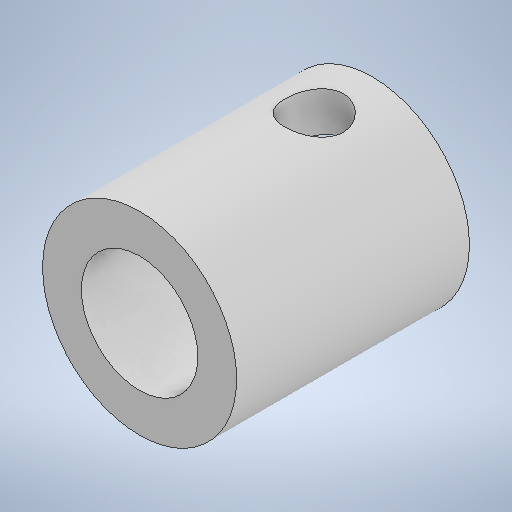
# Autodesk Inventor part: entretoise moteur cremaillere
Saved by Autodesk Inventor 2025.2 (Build 292293000, 293)
## iProperties
Created: 2025-03-30
Part Number: entretoise moteur cremaillere
Material: Générique
Document SubType Name: Modeling
Designer: enezl
Density: 1 g/cm^3
Appearance: Par défaut
Author: enezl
Autodesk Inventor part; units mm, degrees
ref_plane "YZ Plane" through (0, 0, 0) normal (1, 0, 0) x (0, 1, 0)
ref_plane "XY Plane" through (0, 0, 0) normal (0, 0, 1) x (1, 0, 0)
sketch "Esquisse1" plane through (0, 0, 0) normal (1, 0, 0) x (0, 1, 0)
  line L0 (5, 6) -> (3, 6)
  line L1 (3, 6) -> (3, -6)
  line L2 (3, -6) -> (5, -6)
  line L3 (5, -6) -> (5, 6)
  line L4 (5, 6) -> (3, -6) construction
  line L5 (3, 6) -> (5, -6) construction
  line L6 (0, 12.4388) -> (0, -12.4388)
  line L7 (0, 0) -> (14.0159, 0) construction
  point P0 (4, 0)
  dimension "d0" = 6
  dimension "d1" = 10
  dimension "d2" = 12
  constraints: 16 end point, 3 midpoint, 2 horizontal, 2 parallel, 1 coincident, 1 perpendicular, 1 point on line, 1 vertical
  measures "d0" diameter of L1 L6
  measures "d1" diameter of L3 L6
  measures "d2" distance of L2.end L0.start
revolve "Révolution1" add sketch "Esquisse1" angle 360 about axis through (0, 0, 12.4388) along (0, 0, -1)
ref_plane "Plan de construction1" through (0, 5, 0) normal (0, 1, 0) x (-1, 0, 0)
sketch "Esquisse2" plane through (0, 5, 0) normal (0, 1, 0) x (-1, 0, 0)
  line L0 (0, 0) -> (0, -3) construction
  dimension "d4" = 3
  constraints: 2 end point, 1 vertical
  measures "d4" distance of L0.start L0.end
hole "Perçage1" at (0, 5, -3) direction (0, -1, 0) diameter 3 end up to face face through (0, 0, 0) facing (0, 0, -1) round with radius 3 far side yes
